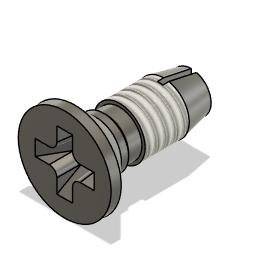
final_combined_updated (Autodesk Fusion 360 archive; units mm, degrees)
design "Type I Cross Recessed Flat Countersunk Head Tapping Screw ASME B18.6.5M M2.5x0.45 x 6 Type D Steel Grade 2 Plain"
description: Type I Cross Recessed Flat Countersunk Head Tapping Screw ASME B18.6.5M M2.5x0.45 x 6 Type D
part number: CRFCHTS ASME B18.6.5M - M2.5x0.45 x 6 - D - I Steel Grade 2 Plain
Autodesk Fusion 360 part; units mm, degrees
sketch "Sketch1" plane through (0, 0, 0) normal (0, 1, 0) x (1, 0, 0)
  line L0 (0, -2.68) -> (-2.2, -2.68)
  line L1 (-2.2, -2.68) -> (-2.2, -2.2)
  line L2 (-2.2, -2.2) -> (-1.18, -1.18)
  line L3 (-1.18, -1.18) -> (0, 0) construction
  line L4 (-1.25, 3.32) -> (0, 3.32)
  line L5 (0, 3.32) -> (0, -2.68)
  line L6 (-1.18, -1.18) -> (-1.18, -0.83)
  line L7 (-1.18, -0.83) -> (-1.0625, -0.7125)
  line L8 (-1.0625, -0.7125) -> (-1.0625, -0.08)
  line L9 (-1.0625, -0.08) -> (-1.25, -0.08)
  line L10 (-1.25, -0.08) -> (-1.25, 3.32)
  line L11 (-1.18, -1.18) -> (0, -1.18) construction
  dimension "d5" = 45
  dimension "d9" = 2.5
  dimension "d11" = 4.4
  dimension "d68" = 1.5
  dimension "d94" = 3.4
  dimension "d95" = 2.125
  dimension "d96" = 45
  dimension "d97" = 2.36
  dimension "d102" = 6
  dimension "d103" = 0.35
  constraint perpendicular L0 L1
  constraint collinear L2 L3
  constraint perpendicular L0 L5
  constraint collinear L3.end L0.start L4.end
  constraint coincident L3.end L5
  constraint coincident origin L3
  constraint horizontal L0
  constraint vertical L6
  constraint parallel L6 L8
  constraint perpendicular L8 L9
  constraint perpendicular L4 L10
  constraint vertical L10
  constraint coincident L5 L11.end
  constraint perpendicular L5 L11
  measures "d5" angle of L3 L5
  measures "d68" distance of L0 L2.end
  measures "d94" distance of L4 L9
  measures "d96" angle of L6 L7
  measures "d102" distance of L0.start L4
  measures "d103" distance of L6.end L11
revolve "Revolve1" add sketch "Sketch1" angle 360 about axis through (0, 0, -3.32) along (0, 0, 1) makes body 1
sketch "Sketch2" plane through (0, 0, 2.68) normal (0, 0, 1) x (1, 0, 0)
  line L0 (-0.37, 0.37) -> (-1.4, 0.37)
  line L1 (-1.4, 0.37) -> (-1.4, -0.37)
  line L2 (-1.4, -0.37) -> (-0.37, -0.37)
  line L3 (-0.37, -0.37) -> (-0.37, -1.4)
  line L4 (-0.37, -1.4) -> (0.37, -1.4)
  line L5 (0.37, -1.4) -> (0.37, -0.37)
  line L6 (0.37, -0.37) -> (1.4, -0.37)
  line L7 (1.4, -0.37) -> (1.4, 0.37)
  line L8 (1.4, 0.37) -> (0.37, 0.37)
  line L9 (0.37, 0.37) -> (0.37, 1.4)
  line L10 (0.37, 1.4) -> (-0.37, 1.4)
  line L11 (-0.37, 1.4) -> (-0.37, 0.37)
  dimension "d104" = 0.74
  dimension "d106" = 360
  dimension "d107" = 2.8
  constraint horizontal L0
  constraint perpendicular L0 L1
  constraint horizontal L2
  constraint vertical L0.start L2.end
  constraint coincident L0.start L11.end
  measures "d104" distance of L0 L1.end
  measures "d107" distance of L3.end L10
extrude "Extrude1" add sketch "Sketch2" against normal blind 1.78 draft -4 separate body makes body 2
draft "Draft1" angle -30 neutral plane through (0, 0, 2.68) pull (0, 0, 1) 4 faces at (1.3585, 0.0818, 2.0867) (-0.0818, 1.3585, 2.0867) (-0.0818, -1.3585, 2.0867) (-1.3585, 0.0818, 2.0867) on bodies 2
fillet "Fillet3" radius 0.364 4 edges at (0.3078, 0.3078, 1.79) (-0.3078, 0.3078, 1.79) (-0.3078, -0.3078, 1.79) (0.3078, -0.3078, 1.79) on bodies 2
combine "Combine1" operation cut target body 1 tool bodies 2
thread "Thread1" "ANSI Metric M Profile 2.5 M2.5x0.45 6g" major diameter 2.43 minor diameter 1.9165 pitch 0.45 angle 60 resizes the face on face at (-1.2484, 0.0623, -1.0533) on bodies 1
sketch "Sketch5" plane through (0, 0, 0) normal (0, 1, 0) x (1, 0, 0)
  line L0 (-1.275, 3.32) -> (-1.275, 1.72)
  line L1 (-1.275, 1.72) -> (-0.94, 3.32)
  line L2 (0, 3.32) -> (0, -2.68)
  line L3 (0, 3.32) -> (-1.275, 3.32)
  dimension "d81" = 1.275
  dimension "d110" = 0.94
  dimension "d111" = 1.6
  constraint vertical L0
  constraint coincident L2.start L3.start
  constraint perpendicular L0 L3
  constraint coincident L1.end L3
  measures "d81" distance of origin L0
  measures "d110" distance of L1.end L2
  measures "d111" distance of L0.end L3
revolve "Revolve2" cut sketch "Sketch5" angle 360 about axis through (0, 0, -3.32) along (0, 0, 1) bodies 1
sketch "Sketch6" plane through (0, 0, -3.32) normal (0, 0, -1) x (-1, 0, 0)
  line L0 (-0.25, 2.2) -> (0, 2.2)
  line L1 (0, 2.2) -> (0, 0)
  line L2 (0, 0) -> (-0.25, 0)
  circle A0 centre (0, 0) radius 0.94
  line L3 (-0.25, 2.2) -> (-0.25, 0)
  dimension "d112" = 0.25
  dimension "d113" = 2.2
  constraint horizontal L2
  constraint coincident L1.end L2.start
  constraint perpendicular L1 L2
  constraint perpendicular L0 L1
  constraint perpendicular L0 L3
  measures "d112" distance of L0.end L3
  measures "d113" distance of L1.end L0
extrude "Extrude2" cut sketch "Sketch6" against normal blind 1.6 contours L0 L1 A0 L3 | L1 L2 A0 L3 picked at (-0.1667, 0.302) bodies 1
equation "d5 = adsk_headang * 0.5"
equation "d9 = adsk_nomdia"
equation "d11 = adsk_headdia"
equation "adsk_nomlen = 6.00 mm"
equation "adsk_headh = 1.50 mm"
equation "adsk_headdia = 4.40 mm"
equation "adsk_nomdia = 2.50 mm"
equation "adsk_headang = 90.00 deg"
equation "adsk_phildia = 2.80 mm"
equation "d31 = -adsk_phildepth"
equation "adsk_philwidth = 0.74 mm"
equation "adsk_phildepth = 1.78 mm"
equation "adsk_startlen = 1.60 mm"
equation "d68 = adsk_headh"
equation "d73 = -adsk_startlen"
equation "adsk_endpointdia = 1.88 mm"
equation "d81 = adsk_nomdia * 0.51"
equation "d86 = ( adsk_nomdia * 0.5 ) * tan(90 deg - adsk_headang * 0.5) + adsk_headh"
equation "adsk_thrlen = 3.40 mm"
equation "adsk_grpdia = 2.36 mm"
equation "adsk_grplen = 0.35 mm"
equation "adsk_shlang = 45.00 deg"
equation "d94 = adsk_thrlen"
equation "d95 = adsk_shnkdia"
equation "d96 = adsk_shlang"
equation "d97 = adsk_grpdia"
equation "adsk_shnkdia = adsk_nomdia * 0.85"
equation "d102 = adsk_nomlen"
equation "d103 = adsk_grplen"
equation "d104 = adsk_philwidth"
equation "d107 = adsk_phildia"
equation "d109 = adsk_phildia * 0.13"
equation "d110 = adsk_endpointdia / 2"
equation "d111 = adsk_startlen"
equation "d112 = adsk_nomdia / 10"
equation "d113 = adsk_headdia / 2"

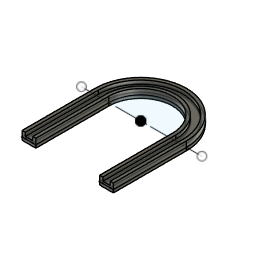
design "supporter"
Autodesk Fusion 360 part; units mm, degrees
sketch "Sketch1" plane through (0, 0, 0) normal (0, 0, 1) x (1, 0, 0)
  line L0 (-65, 0) -> (67.0686, 0)
  line L1 (-35, 0) -> (-35, -80)
  line L2 (-50, 0) -> (-50, -80)
  line L3 (35, 0) -> (35, -80)
  line L4 (50, 0) -> (50, -80)
  line L5 (35, -80) -> (50, -80)
  line L6 (-50, -80) -> (-35, -80)
  arc A0 (35, 0) -> (-35, 0) centre (0, 0) ccw
  arc A1 (50, 0) -> (-50, 0) centre (0, 0) ccw
  arc A2 (38.5, 0) -> (-38.5, 0) centre (0, 0) ccw
  arc A3 (46.5, 0) -> (-46.5, 0) centre (0, 0) ccw
  line L7 (-38.5, 0) -> (-38.5, -80)
  line L8 (-46.5, 0) -> (-46.5, -80)
  line L9 (38.5, 0) -> (38.5, -80)
  line L10 (46.5, 0) -> (46.5, -80)
  dimension "d1" = 70
  dimension "d2" = 100
  dimension "d3" = 80
  dimension "d4" = 80
  dimension "d5" = 80
  dimension "d8" = 77
  dimension "d9" = 93
  constraint coincident A0.centre A1.centre
  constraint horizontal L0
  constraint coincident L0 L1.start
  constraint tangent L1 A0
  constraint perpendicular L0 L1
  constraint coincident L0 L2.start
  constraint tangent L2 A1
  constraint coincident L0 L3.start
  constraint tangent L3 A0
  constraint coincident L0 L4.start
  constraint tangent L4 A1
  constraint perpendicular L4 L5
  constraint concentric A0 A3
  constraint coincident L0 A2.end
  constraint coincident L0 A2.start
  constraint coincident L0 A3.end
  constraint coincident L0 A3.start
  constraint coincident L6 L7.end
  constraint tangent A2 L7
  constraint coincident L6 L8.end
  constraint tangent A3 L8
  constraint coincident L5 L9.end
  constraint tangent A2 L9
  constraint coincident L5 L10.end
  constraint tangent A3 L10
  measures "d1" diameter of A0
  measures "d2" diameter of A1
  measures "d3" distance of L1.start L1.end
  measures "d4" distance of L2.start L2.end
  measures "d5" distance of L4.start L4.end
  measures "d8" diameter of A2
  measures "d9" diameter of A3
extrude "Extrude2" add sketch "Sketch1" along normal blind 6 contours L0 A1 A3 | L0 L2 L6 L8 | L0 L4 L5 L10 | L0 A0 A2 | L0 L1 L6 L7 | L0 L3 L5 L9 makes body 1 at (36.1667, -53.3333, 0) makes body 2 at (-47.6667, -53.3333, 0)
extrude "Extrude3" add sketch "Sketch1" along normal blind 2 separate body contours L0 A2 A3 | L0 L6 L7 L8 | L0 L5 L9 L10 makes body 3
extrude "Extrude4" add sketch "Sketch1" against normal blind 3.3 contours L0 A1 A3 | L0 L2 L6 L8 | L0 A2 A3 | L0 L6 L7 L8 | L0 L4 L5 L10 | L0 A0 A2 | L0 L1 L6 L7 | L0 L5 L9 L10 | L0 L3 L5 L9 bodies 1 2 3
